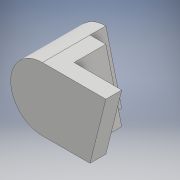
# Autodesk Inventor part: 6
Saved by Autodesk Inventor 2017 (Build 210142000, 142)
## iProperties
Part Number: 6
Material: 一般
Document SubType Name: Modeling
Designer: Brian
Density: 1 g/cm^3
Appearance: 預設
Author: Brian
Autodesk Inventor part; units mm, degrees
ref_plane "YZ Plane" through (0, 0, 0) normal (1, 0, 0) x (0, 1, 0)
ref_plane "XZ Plane" through (0, 0, 0) normal (0, 1, 0) x (-1, 0, 0)
ref_plane "XY Plane" through (0, 0, 0) normal (0, 0, 1) x (1, 0, 0)
sketch "草圖1" plane through (0, 0, 0) normal (0, 1, 0) x (-1, 0, 0)
  line L0 (0, 0) -> (0, -40)
  line L1 (0, -40) -> (-50, -40)
  line L2 (0, 0) -> (-60, 0)
  line L3 (-60, 0) -> (-50, -40)
  dimension "d0" = 60
  dimension "d1" = 40
  dimension "d2" = 50
  constraints: 8 end point, 2 horizontal, 1 vertical
  measures "d0" distance of L0.start L2.end
  measures "d1" vertical distance of L2.end L1.end
  measures "d2" distance of L0.end L1.end
extrude "擠出1" add sketch "草圖1" along normal blind 10
sketch "草圖2" plane through (0, 10, 0) normal (0, 1, 0) x (1, 0, 0)
  line L0 (50, 40) -> (0, 40) projected
  line L1 (40, 40) -> (30, 0)
  line L2 (30, 0) -> (0, 0)
  line L3 (0, 0) -> (0, 40)
  line L4 (0, 40) -> (0, 0) projected
  line L5 (0, 40) -> (40, 40)
  dimension "d5" = 10
  dimension "d6" = 10
  constraints: 8 end point, 1 horizontal, 1 parallel, 1 perpendicular, 1 point on line
  measures "d5" distance of L0.start L1.start
  measures "d6" horizontal distance of L1.start L1.end
extrude "擠出2" add sketch "草圖2" along normal blind 20
sketch "草圖3" plane through (0, 30, 0) normal (0, 1, 0) x (1, 0, 0)
  line L0 (30, 0) -> (40, 40) projected
  line L1 (20, 0) -> (30, 40)
  line L2 (30, 40) -> (0, 40)
  line L3 (0, 0) -> (0, 40) projected
  line L4 (0, 40) -> (0, 0)
  line L5 (0, 0) -> (20, 0)
  line L6 (60, 0) -> (0, 0) projected
  dimension "d9" = 10
  dimension "d10" = 10
  constraints: 8 end point, 1 collinear, 1 horizontal, 1 perpendicular
  measures "d9" distance of L0.start L1.start
  measures "d10" distance of L0.end L1.end
extrude "擠出3" add sketch "草圖3" along normal blind 10
fillet "圓角1" radius 20 2 edges at (0, 20, 0) (0, 20, -40)
